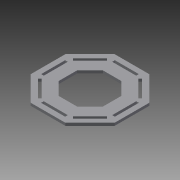
# Autodesk Inventor part: octoBotoStemRingLarger01
Saved by Autodesk Inventor 2013 (Build 170138000, 138)
## iProperties
Created: 2014-11-13
Part Number: octoBotoStemRingLarger01
Material: Generic
Document SubType Name: Modeling
Designer: Nano
Density: 1 g/cm^3
Author: Nano
Autodesk Inventor part; units mm, degrees
ref_plane "YZ Plane" through (0, 0, 0) normal (1, 0, 0) x (0, 1, 0)
ref_plane "XZ Plane" through (0, 0, 0) normal (0, 1, 0) x (-1, 0, 0)
ref_plane "XY Plane" through (0, 0, 0) normal (0, 0, 1) x (1, 0, 0)
sketch "Sketch1" plane through (0, 0, 0) normal (0, 1, 0) x (-1, 0, 0)
  line L0 (-14.2875, -40.7478) -> (14.2875, -40.7478)
  line L1 (14.2875, -40.7478) -> (14.2875, -43.9228)
  line L2 (14.2875, -43.9228) -> (-14.2875, -43.9228)
  line L3 (-14.2875, -43.9228) -> (-14.2875, -40.7478)
  line L4 (18.7102, -38.9158) -> (38.9158, -18.7102)
  line L5 (38.9158, -18.7102) -> (41.1609, -20.9553)
  line L6 (41.1609, -20.9553) -> (20.9553, -41.1609)
  line L7 (20.9553, -41.1609) -> (18.7102, -38.9158)
  line L8 (40.7478, -14.2875) -> (40.7478, 14.2875)
  line L9 (40.7478, 14.2875) -> (43.9228, 14.2875)
  line L10 (43.9228, 14.2875) -> (43.9228, -14.2875)
  line L11 (43.9228, -14.2875) -> (40.7478, -14.2875)
  line L12 (38.9158, 18.7102) -> (18.7102, 38.9158)
  line L13 (18.7102, 38.9158) -> (20.9553, 41.1609)
  line L14 (20.9553, 41.1609) -> (41.1609, 20.9553)
  line L15 (41.1609, 20.9553) -> (38.9158, 18.7102)
  line L16 (14.2875, 40.7478) -> (-14.2875, 40.7478)
  line L17 (-14.2875, 40.7478) -> (-14.2875, 43.9228)
  line L18 (-14.2875, 43.9228) -> (14.2875, 43.9228)
  line L19 (14.2875, 43.9228) -> (14.2875, 40.7478)
  line L20 (-18.7102, 38.9158) -> (-38.9158, 18.7102)
  line L21 (-38.9158, 18.7102) -> (-41.1609, 20.9553)
  line L22 (-41.1609, 20.9553) -> (-20.9553, 41.1609)
  line L23 (-20.9553, 41.1609) -> (-18.7102, 38.9158)
  line L24 (-40.7478, 14.2875) -> (-40.7478, -14.2875)
  line L25 (-40.7478, -14.2875) -> (-43.9228, -14.2875)
  line L26 (-43.9228, -14.2875) -> (-43.9228, 14.2875)
  line L27 (-43.9228, 14.2875) -> (-40.7478, 14.2875)
  line L28 (-38.9158, -18.7102) -> (-18.7102, -38.9158)
  line L29 (-18.7102, -38.9158) -> (-20.9553, -41.1609)
  line L30 (-20.9553, -41.1609) -> (-41.1609, -20.9553)
  line L31 (-41.1609, -20.9553) -> (-38.9158, -18.7102)
  line L32 (50.0728, -20.7409) -> (20.7409, -50.0728)
  line L33 (20.7409, -50.0728) -> (-20.7409, -50.0728)
  line L34 (-20.7409, -50.0728) -> (-50.0728, -20.7409)
  line L35 (-50.0728, -20.7409) -> (-50.0728, 20.7409)
  line L36 (-50.0728, 20.7409) -> (-20.7409, 50.0728)
  line L37 (-20.7409, 50.0728) -> (20.7409, 50.0728)
  line L38 (20.7409, 50.0728) -> (50.0728, 20.7409)
  line L39 (50.0728, 20.7409) -> (50.0728, -20.7409)
  line L40 (26.3506, -10.9148) -> (10.9148, -26.3506)
  line L41 (10.9148, -26.3506) -> (-10.9148, -26.3506)
  line L42 (-10.9148, -26.3506) -> (-26.3506, -10.9148)
  line L43 (-26.3506, -10.9148) -> (-26.3506, 10.9148)
  line L44 (-26.3506, 10.9148) -> (-10.9148, 26.3506)
  line L45 (-10.9148, 26.3506) -> (10.9148, 26.3506)
  line L46 (10.9148, 26.3506) -> (26.3506, 10.9148)
  line L47 (26.3506, 10.9148) -> (26.3506, -10.9148)
  point P0 (0, 0)
  point P1 (0, 0)
  point P2 (0, 0)
  point P3 (0, 0)
  dimension "d0" = 28.575
  dimension "d1" = 3.175
  dimension "d2" = 43.18
  dimension "d3" = 43.18
  dimension "d6" = 360
  constraints: 96 end point, 4 parallel, 1 horizontal, 1 perpendicular, 99 other
  measures "d0" distance of L1.end L2.end
  measures "d1" distance of L0.end L1.end
  measures "d2" distance of point (0, 0) L0.start
  measures "d3" distance of L0.end point (0, 0)
extrude "Extrusion1" add sketch "Sketch1" along normal blind 3.175
equation "\"d3\" = d2"
body "Solid1"
